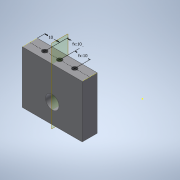
# Autodesk Inventor part: Y screw bracket
Saved by Autodesk Inventor 2020 (Build 240168000, 168)
## iProperties
Created: 2019-02-27
Part Number: Y screw bracket
Material: Generic
Document SubType Name: Modeling
Designer: LillaHunden
Density: 1 g/cm^3
Appearance: Default
Author: LillaHunden
Autodesk Inventor part; units mm, degrees
ref_plane "YZ Plane" through (0, 0, 0) normal (1, 0, 0) x (0, 1, 0)
ref_plane "XZ Plane" through (0, 0, 0) normal (0, 1, 0) x (-1, 0, 0)
ref_plane "XY Plane" through (0, 0, 0) normal (0, 0, 1) x (1, 0, 0)
sketch "Sketch1" plane through (0, 0, 0) normal (0, 0, 1) x (1, 0, 0)
  line L0 (-30.1791, 10) -> (-70.1791, 10)
  line L1 (-70.1791, 10) -> (-70.1791, 45)
  line L2 (-70.1791, 45) -> (-30.1791, 45)
  line L3 (-30.1791, 45) -> (-30.1791, 10)
  point P0 (0, 0)
  dimension "d0" = 40
  dimension "d1" = 35
  constraints: 8 end point, 2 parallel, 1 horizontal, 1 perpendicular
  measures "d0" distance of L1.end L2.end
  measures "d1" distance of L0.end L1.end
extrude "Extrusion1" add sketch "Sketch1" along normal blind 10
ref_plane "Work Plane1" through (-50.1791, 10, 0) normal (-1, 0, 0) x (0, 0, 1)
sketch "Sketch2" plane through (0, 0, 0) normal (0, 0, -1) x (-1, 0, 0)
  circle A0 centre (50.1791, 23) radius 4.5 projected
  point P0 (0, 0)
extrude "Extrusion2" cut sketch "Sketch2" against normal through all
sketch "Sketch3" plane through (0, 0, 0) normal (0, 0, -1) x (-1, 0, 0)
  circle A0 centre (50.1791, 23) radius 11 construction
  spline S0 degree 3 poles (51.7186, 14.1946) (51.5683, 14.2588) (51.4334, 14.3531) (51.3179, 14.4692) (51.3108, 14.4763) (51.3038, 14.4836) (51.2968, 14.4909) (51.1938, 14.5992) (51.109, 14.7236) (51.0458, 14.8586) (51.0386, 14.8738) (51.0318, 14.8892) (51.0252, 14.9047) (51.0208, 14.915) (51.0166, 14.9253) (51.0125, 14.9356) (50.9793, 15.0198) (50.9546, 15.1068) (50.9393, 15.1954) (50.93, 15.2495) (50.9242, 15.3043) (50.9217, 15.3594) (50.9209, 15.3759) (50.9205, 15.3925) (50.9204, 15.409) (50.9202, 15.4243) (50.9204, 15.4397) (50.9207, 15.455) (50.9244, 15.605) (50.952, 15.7541) (51.0007, 15.897) (51.007, 15.9155) (51.0136, 15.9339) (51.0207, 15.9522) (51.0249, 15.9632) (51.0292, 15.9741) (51.0337, 15.9851) (51.0715, 16.0773) (51.1181, 16.1657) (51.1728, 16.2486) (51.1817, 16.2621) (51.1908, 16.2754) (51.2001, 16.2886) (51.207, 16.2983) (51.2139, 16.3079) (51.221, 16.3174) (51.2572, 16.3662) (51.2964, 16.4127) (51.3383, 16.4565) (51.3579, 16.477) (51.3782, 16.4969) (51.399, 16.5162) (51.4169, 16.5328) (51.4352, 16.5488) (51.4557, 16.5626) knots 0 0 0 0 0.171917 0.171917 0.171917 0.182531 0.182531 0.182531 0.339556 0.339556 0.339556 0.35729 0.35729 0.35729 0.369023 0.369023 0.369023 0.464442 0.464442 0.464442 0.522742 0.522742 0.522742 0.540193 0.540193 0.540193 0.556325 0.556325 0.556325 0.714368 0.714368 0.714368 0.734813 0.734813 0.734813 0.747126 0.747126 0.747126 0.851246 0.851246 0.851246 0.868176 0.868176 0.868176 0.880588 0.880588 0.880588 0.944403 0.944403 0.944403 0.974326 0.974326 0.974326 1 1 1 1 construction
  arc A1 (53.4951, 16.3178) -> (51.4555, 16.5624) centre (52.3382, 15.2969) ccw construction
  spline S1 degree 3 poles (53.4951, 16.3178) (53.6087, 16.1634) (53.6902, 15.988) (53.738, 15.8022) (53.7411, 15.7901) (53.7441, 15.7778) (53.7469, 15.7656) (53.7877, 15.5892) (53.7975, 15.4072) (53.7737, 15.2288) (53.7723, 15.2187) (53.7709, 15.2087) (53.7693, 15.1987) (53.755, 15.1067) (53.7316, 15.0168) (53.6988, 14.9302) (53.6793, 14.8789) (53.6565, 14.8287) (53.6307, 14.7799) (53.6227, 14.7649) (53.6144, 14.7499) (53.6058, 14.7351) (53.5982, 14.7222) (53.5905, 14.7093) (53.5825, 14.6965) (53.4949, 14.5565) (53.3824, 14.4325) (53.2512, 14.3311) (53.2424, 14.3243) (53.2336, 14.3176) (53.2246, 14.311) (53.1543, 14.2593) (53.0794, 14.2144) (53.0008, 14.1775) (52.9897, 14.1723) (52.9786, 14.1672) (52.9673, 14.1623) (52.8938, 14.1303) (52.8177, 14.1054) (52.7396, 14.0885) (52.72, 14.0843) (52.7002, 14.0806) (52.6795, 14.0793) knots 0 0 0 0 0.200829 0.200829 0.200829 0.213978 0.213978 0.213978 0.403633 0.403633 0.403633 0.414319 0.414319 0.414319 0.512539 0.512539 0.512539 0.570815 0.570815 0.570815 0.588808 0.588808 0.588808 0.60461 0.60461 0.60461 0.77833 0.77833 0.77833 0.789949 0.789949 0.789949 0.881423 0.881423 0.881423 0.894318 0.894318 0.894318 0.978751 0.978751 0.978751 1 1 1 1 construction
  arc A2 (51.7186, 14.1946) -> (52.6795, 14.0793) centre (52.3382, 15.2969) ccw construction
  spline S2 degree 3 poles (57.2626, 24.0568) (57.1288, 24.114) (57.0072, 24.1951) (56.9006, 24.294) (56.8875, 24.3062) (56.8746, 24.3187) (56.862, 24.3314) (56.8548, 24.3386) (56.8478, 24.3458) (56.8408, 24.3532) (56.7378, 24.4615) (56.653, 24.5859) (56.5898, 24.7208) (56.5826, 24.7361) (56.5758, 24.7515) (56.5692, 24.767) (56.5649, 24.7772) (56.5606, 24.7875) (56.5565, 24.7979) (56.5233, 24.8821) (56.4986, 24.969) (56.4833, 25.0577) (56.474, 25.1118) (56.4682, 25.1666) (56.4657, 25.2217) (56.465, 25.2382) (56.4645, 25.2547) (56.4644, 25.2713) (56.4642, 25.2866) (56.4644, 25.3019) (56.4647, 25.3172) (56.4689, 25.4867) (56.5035, 25.655) (56.5647, 25.8144) (56.5689, 25.8254) (56.5732, 25.8364) (56.5777, 25.8473) (56.6155, 25.9396) (56.6621, 26.0279) (56.7168, 26.1109) (56.7257, 26.1244) (56.7348, 26.1377) (56.7441, 26.1509) (56.751, 26.1606) (56.7579, 26.1701) (56.765, 26.1796) (56.8183, 26.2514) (56.8777, 26.318) (56.943, 26.3784) (56.9609, 26.395) (56.9792, 26.4111) (56.9997, 26.4248) knots 0 0 0 0 0.153066 0.153066 0.153066 0.171917 0.171917 0.171917 0.182531 0.182531 0.182531 0.339556 0.339556 0.339556 0.35729 0.35729 0.35729 0.369023 0.369023 0.369023 0.464442 0.464442 0.464442 0.522742 0.522742 0.522742 0.540193 0.540193 0.540193 0.556325 0.556325 0.556325 0.734813 0.734813 0.734813 0.747126 0.747126 0.747126 0.851246 0.851246 0.851246 0.868176 0.868176 0.868176 0.880588 0.880588 0.880588 0.974326 0.974326 0.974326 1 1 1 1 construction
  arc A3 (59.0391, 26.1801) -> (56.9995, 26.4247) centre (57.8822, 25.1591) ccw construction
  spline S3 degree 3 poles (59.0391, 26.1801) (59.1386, 26.0448) (59.2134, 25.8935) (59.2626, 25.7333) (59.2696, 25.7105) (59.276, 25.6876) (59.282, 25.6645) (59.2851, 25.6523) (59.2881, 25.6401) (59.2909, 25.6279) (59.3268, 25.4728) (59.3387, 25.3134) (59.3249, 25.156) (59.323, 25.1343) (59.3206, 25.1127) (59.3177, 25.091) (59.3163, 25.081) (59.3149, 25.071) (59.3133, 25.061) (59.299, 24.969) (59.2756, 24.8791) (59.2428, 24.7925) (59.2233, 24.7411) (59.2006, 24.6909) (59.1747, 24.6422) (59.1667, 24.6271) (59.1584, 24.6122) (59.1498, 24.5974) (59.1423, 24.5844) (59.1345, 24.5715) (59.1265, 24.5588) (59.0486, 24.4343) (58.951, 24.3225) (58.8381, 24.2279) (58.8241, 24.2161) (58.8098, 24.2046) (58.7952, 24.1933) (58.7864, 24.1865) (58.7776, 24.1798) (58.7686, 24.1733) (58.6983, 24.1215) (58.6234, 24.0767) (58.5448, 24.0397) (58.5337, 24.0345) (58.5226, 24.0294) (58.5113, 24.0246) (58.4379, 23.9926) (58.3617, 23.9677) (58.2836, 23.9508) (58.264, 23.9465) (58.2442, 23.9428) (58.2235, 23.9415) knots 0 0 0 0 0.175859 0.175859 0.175859 0.200829 0.200829 0.200829 0.213978 0.213978 0.213978 0.380655 0.380655 0.380655 0.403633 0.403633 0.403633 0.414319 0.414319 0.414319 0.512539 0.512539 0.512539 0.570815 0.570815 0.570815 0.588808 0.588808 0.588808 0.60461 0.60461 0.60461 0.759068 0.759068 0.759068 0.77833 0.77833 0.77833 0.789949 0.789949 0.789949 0.881423 0.881423 0.881423 0.894318 0.894318 0.894318 0.978751 0.978751 0.978751 1 1 1 1 construction
  arc A4 (57.2626, 24.0568) -> (58.2235, 23.9415) centre (57.8822, 25.1591) ccw construction
  spline S4 degree 3 poles (47.4003, 29.6009) (47.2501, 29.665) (47.1151, 29.7593) (46.9997, 29.8754) (46.9926, 29.8826) (46.9855, 29.8898) (46.9786, 29.8972) (46.8755, 30.0055) (46.7907, 30.1299) (46.7275, 30.2649) (46.7204, 30.2801) (46.7135, 30.2955) (46.707, 30.311) (46.7026, 30.3212) (46.6984, 30.3316) (46.6943, 30.3419) (46.661, 30.4261) (46.6364, 30.513) (46.6211, 30.6017) (46.6118, 30.6558) (46.6059, 30.7106) (46.6035, 30.7657) (46.6027, 30.7822) (46.6023, 30.7987) (46.6021, 30.8153) (46.602, 30.8306) (46.6021, 30.8459) (46.6025, 30.8612) (46.6066, 31.0307) (46.6413, 31.199) (46.7024, 31.3584) (46.7066, 31.3694) (46.711, 31.3804) (46.7155, 31.3913) (46.7533, 31.4836) (46.7999, 31.5719) (46.8546, 31.6549) (46.8635, 31.6684) (46.8726, 31.6817) (46.8819, 31.6949) (46.8887, 31.7046) (46.8957, 31.7142) (46.9027, 31.7237) (46.956, 31.7954) (47.0155, 31.862) (47.0808, 31.9225) (47.0986, 31.939) (47.117, 31.9551) (47.1374, 31.9688) knots 0 0 0 0 0.171917 0.171917 0.171917 0.182531 0.182531 0.182531 0.339556 0.339556 0.339556 0.35729 0.35729 0.35729 0.369023 0.369023 0.369023 0.464442 0.464442 0.464442 0.522742 0.522742 0.522742 0.540193 0.540193 0.540193 0.556325 0.556325 0.556325 0.734813 0.734813 0.734813 0.747125 0.747125 0.747125 0.851246 0.851246 0.851246 0.868176 0.868176 0.868176 0.880588 0.880588 0.880588 0.974325 0.974325 0.974325 1 1 1 1 construction
  arc A5 (49.1769, 31.7241) -> (47.1373, 31.9687) centre (48.02, 30.7031) ccw construction
  spline S5 degree 3 poles (49.1769, 31.7241) (49.2763, 31.5889) (49.3511, 31.4376) (49.4003, 31.2773) (49.4073, 31.2545) (49.4138, 31.2316) (49.4197, 31.2085) (49.4229, 31.1963) (49.4258, 31.1841) (49.4287, 31.1719) (49.4695, 30.9954) (49.4793, 30.8134) (49.4554, 30.6351) (49.4541, 30.625) (49.4526, 30.615) (49.4511, 30.605) (49.4367, 30.513) (49.4134, 30.4231) (49.3806, 30.3365) (49.3551, 30.2693) (49.3239, 30.2041) (49.2875, 30.1414) (49.28, 30.1284) (49.2722, 30.1155) (49.2643, 30.1028) (49.1864, 29.9783) (49.0888, 29.8665) (48.9759, 29.7719) (48.9618, 29.7601) (48.9475, 29.7486) (48.933, 29.7373) (48.9242, 29.7305) (48.9153, 29.7239) (48.9064, 29.7173) (48.8361, 29.6656) (48.7612, 29.6207) (48.6826, 29.5837) (48.6715, 29.5785) (48.6603, 29.5735) (48.6491, 29.5686) (48.5756, 29.5366) (48.4995, 29.5117) (48.4214, 29.4948) (48.4017, 29.4906) (48.382, 29.4868) (48.3612, 29.4855) knots 0 0 0 0 0.175859 0.175859 0.175859 0.200829 0.200829 0.200829 0.213978 0.213978 0.213978 0.403633 0.403633 0.403633 0.414319 0.414319 0.414319 0.512539 0.512539 0.512539 0.588808 0.588808 0.588808 0.60461 0.60461 0.60461 0.759068 0.759068 0.759068 0.77833 0.77833 0.77833 0.789949 0.789949 0.789949 0.881423 0.881423 0.881423 0.894318 0.894318 0.894318 0.978751 0.978751 0.978751 1 1 1 1 construction
  arc A6 (47.4003, 29.6009) -> (48.3612, 29.4855) centre (48.02, 30.7031) ccw construction
  spline S6 degree 3 poles (41.8563, 19.7386) (41.7225, 19.7957) (41.6009, 19.8768) (41.4944, 19.9758) (41.4812, 19.988) (41.4683, 20.0005) (41.4557, 20.0132) (41.4486, 20.0203) (41.4415, 20.0276) (41.4345, 20.0349) (41.3315, 20.1433) (41.2467, 20.2677) (41.1835, 20.4026) (41.1764, 20.4178) (41.1695, 20.4332) (41.1629, 20.4487) (41.1586, 20.459) (41.1544, 20.4693) (41.1503, 20.4797) (41.117, 20.5638) (41.0924, 20.6508) (41.0771, 20.7394) (41.0678, 20.7936) (41.0619, 20.8483) (41.0594, 20.9034) (41.0587, 20.9199) (41.0583, 20.9365) (41.0581, 20.953) (41.058, 20.9683) (41.0581, 20.9837) (41.0585, 20.999) (41.0626, 21.1685) (41.0972, 21.3367) (41.1584, 21.4962) (41.1626, 21.5072) (41.167, 21.5182) (41.1714, 21.5291) (41.2154, 21.6364) (41.2712, 21.7383) (41.3379, 21.8327) (41.3963, 21.9154) (41.4628, 21.9918) (41.5367, 22.0602) (41.5546, 22.0768) (41.5729, 22.0929) (41.5934, 22.1066) knots 0 0 0 0 0.153066 0.153066 0.153066 0.171917 0.171917 0.171917 0.182531 0.182531 0.182531 0.339556 0.339556 0.339556 0.35729 0.35729 0.35729 0.369023 0.369023 0.369023 0.464442 0.464442 0.464442 0.522742 0.522742 0.522742 0.540193 0.540193 0.540193 0.556325 0.556325 0.556325 0.734813 0.734813 0.734813 0.747125 0.747125 0.747125 0.868176 0.868176 0.868176 0.974325 0.974325 0.974325 1 1 1 1 construction
  arc A7 (43.6329, 21.8619) -> (41.5933, 22.1065) centre (42.476, 20.8409) ccw construction
  spline S7 degree 3 poles (43.6329, 21.8619) (43.7464, 21.7074) (43.828, 21.532) (43.8757, 21.3462) (43.8789, 21.3341) (43.8818, 21.3219) (43.8847, 21.3096) (43.9205, 21.1546) (43.9324, 20.9952) (43.9186, 20.8378) (43.9167, 20.8161) (43.9143, 20.7944) (43.9114, 20.7728) (43.9101, 20.7628) (43.9086, 20.7527) (43.907, 20.7427) (43.8927, 20.6508) (43.8693, 20.5608) (43.8365, 20.4743) (43.8171, 20.4229) (43.7943, 20.3727) (43.7684, 20.3239) (43.7604, 20.3089) (43.7521, 20.2939) (43.7435, 20.2792) (43.736, 20.2662) (43.7282, 20.2533) (43.7203, 20.2406) (43.6423, 20.116) (43.5448, 20.0043) (43.4319, 19.9097) (43.4178, 19.8979) (43.4035, 19.8863) (43.3889, 19.8751) (43.3802, 19.8683) (43.3713, 19.8616) (43.3624, 19.855) (43.2921, 19.8033) (43.2172, 19.7584) (43.1385, 19.7215) (43.1275, 19.7163) (43.1163, 19.7112) (43.1051, 19.7063) (43.0316, 19.6743) (42.9555, 19.6494) (42.8774, 19.6326) (42.8577, 19.6283) (42.8379, 19.6246) (42.8172, 19.6233) knots 0 0 0 0 0.200829 0.200829 0.200829 0.213978 0.213978 0.213978 0.380655 0.380655 0.380655 0.403633 0.403633 0.403633 0.414319 0.414319 0.414319 0.512539 0.512539 0.512539 0.570815 0.570815 0.570815 0.588808 0.588808 0.588808 0.60461 0.60461 0.60461 0.759068 0.759068 0.759068 0.77833 0.77833 0.77833 0.789949 0.789949 0.789949 0.881423 0.881423 0.881423 0.894318 0.894318 0.894318 0.978751 0.978751 0.978751 1 1 1 1 construction
  arc A8 (41.8563, 19.7386) -> (42.8172, 19.6233) centre (42.476, 20.8409) ccw construction
  circle A9 centre (50.1791, 23) radius 4.5 construction
  point P0 (0, 0)
hole "Hole1" at (-48.02, 30.7031, 0) at (-42.476, 20.8409, 0) at (-52.3382, 15.2969, 0) at (-57.8822, 25.1591, 0) direction (0, 0, 1) diameter 2.459 end through all thread size "M3x0.5" class "6H" standard "ISO Metric profile"
sketch "Sketch4" plane through (-70.1791, 45, 0) normal (0, 1, 0) x (1, 0, 0)
  line L0 (0, 0) -> (0, -10) construction
  line L1 (0, -5) -> (40, -5) construction
  line L2 (40, 0) -> (40, -10) construction
  point P0 (70.1791, 0)
  point P1 (10, -5)
  point P2 (20, -5)
  point P3 (30, -5)
  dimension "d13" = 10
  dimension "d14" = 10
  dimension "d15" = 10
  constraints: 3 midpoint, 2 end point, 2 point on line
  measures "d13" distance from line of L0 point (10, -5)
  measures "d14" distance of point (20, -5) point (10, -5)
  measures "d15" distance of point (30, -5) point (20, -5)
sketch "Sketch5" plane through (-70.1791, 45, 0) normal (0, 1, 0) x (1, 0, 0)
  point P0 (10, -5)
  point P1 (20, -5)
  point P2 (30, -5)
hole "Hole2" at (-60.1791, 45, 5) at (-50.1791, 45, 5) at (-40.1791, 45, 5) direction (0, -1, 0) diameter 3.242 depth 10 tip angle 120 thread size "M4x0.7" class "6H" standard "ISO Metric profile"
equation "\"d14\" = d13"
equation "\"d15\" = d14"
body "Solid1"
